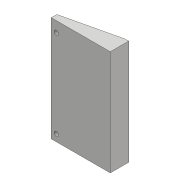
# Autodesk Inventor part: Buck_Bracket
Saved by Autodesk Inventor 2018 (Build 220112000, 112)
## iProperties
Created: 2019-11-08
Part Number: Buck_Bracket
Material: Generic
Document SubType Name: Modeling
Designer: Clevo
Density: 1 g/cm^3
Appearance: Default
Author: Clevo
Autodesk Inventor part; units mm, degrees
ref_plane "YZ Plane" through (0, 0, 0) normal (1, 0, 0) x (0, 1, 0)
ref_plane "XZ Plane" through (0, 0, 0) normal (0, 1, 0) x (-1, 0, 0)
ref_plane "XY Plane" through (0, 0, 0) normal (0, 0, 1) x (1, 0, 0)
sketch "Sketch1" plane through (0, 0, 0) normal (0, 1, 0) x (-1, 0, 0)
  line L0 (-15, -27.5) -> (15, -27.5)
  line L1 (15, -27.5) -> (15, 27.5)
  line L2 (15, 27.5) -> (-15, 27.5)
  line L3 (-15, 27.5) -> (-15, -27.5)
  line L4 (-15, -27.5) -> (15, 27.5) construction
  line L5 (15, -27.5) -> (-15, 27.5) construction
  point P0 (0, 0)
  dimension "d0" = 55
  dimension "d1" = 30
  constraints: 12 end point, 2 midpoint, 2 parallel, 1 horizontal, 1 perpendicular
  measures "d0" distance of L0.end L1.end
  measures "d1" distance of L0.start L0.end
extrude "Extrusion1" add sketch "Sketch1" along normal blind 3
sketch "Sketch2" plane through (0, 3, 0) normal (0, 1, 0) x (1, 0, 0)
  line L0 (10.75, 21.75) -> (-10.75, 21.75)
  line L1 (-10.75, 21.75) -> (-10.75, -21.75)
  line L2 (-10.75, -21.75) -> (10.75, -21.75)
  line L3 (10.75, -21.75) -> (10.75, 21.75)
  line L4 (10.75, 21.75) -> (-10.75, -21.75) construction
  line L5 (-10.75, 21.75) -> (10.75, -21.75) construction
  point P0 (0, 0)
  dimension "d4" = 43.5
  dimension "d5" = 21.5
  constraints: 12 end point, 2 midpoint, 2 parallel, 1 horizontal, 1 perpendicular
  measures "d4" distance of L0.end L1.end
  measures "d5" distance of L1.end L2.end
extrude "Extrusion2" cut sketch "Sketch2" against normal blind 1.6
sketch "Sketch3" plane through (15, 0, 27.5) normal (1, 0, 0) x (0, 0, -1)
  line L0 (55, 0) -> (0, 0) projected
  line L1 (0, 0) -> (55, 0)
  line L2 (55, 0) -> (55, 10)
  line L3 (55, 10) -> (0, 10)
  line L4 (0, 10) -> (0, 0)
  line L5 (55, 0) -> (55, 3) projected
  point P0 (27.5, 0)
  dimension "d8" = 10
  constraints: 8 end point, 2 parallel, 1 collinear, 1 horizontal, 1 perpendicular
  measures "d8" distance of L3.end L0.end
extrude "Extrusion3" add sketch "Sketch3" along normal blind 2
sketch "Sketch4" plane through (-15, 0, 27.5) normal (0, 0, 1) x (1, 0, 0)
  line L0 (0, 0) -> (32, 0) projected
  line L1 (32, 10) -> (32, 0) projected
  line L2 (30, 10) -> (32, 10) projected
  line L3 (30, 10) -> (30, 3) projected
  line L4 (0, 3) -> (30, 3) projected
  line L5 (0, 0) -> (0, 3) projected
  line L6 (0, 3) -> (30, 3) projected
  line L7 (30, 10) -> (32, 10) projected
  line L8 (0, 3) -> (30, 10)
  point P0 (15, 0)
  constraints: 2 end point
extrude "Extrusion4" add sketch "Sketch4" along normal blind 2
sketch "Sketch5" plane through (0, 3, 0) normal (0, 1, 0) x (1, 0, 0)
  line L0 (12.25, 23.75) -> (-12.25, 23.75)
  line L1 (-12.25, 23.75) -> (-12.25, -23.75)
  line L2 (-12.25, -23.75) -> (12.25, -23.75)
  line L3 (12.25, -23.75) -> (12.25, 23.75)
  line L4 (12.25, 23.75) -> (-12.25, -23.75) construction
  line L5 (-12.25, 23.75) -> (12.25, -23.75) construction
  line L6 (-10.75, -21.75) -> (-10.75, 21.75) projected
  line L7 (10.75, -21.75) -> (-10.75, -21.75) projected
  point P0 (0, 0)
  dimension "d13" = 1.5
  dimension "d14" = 2
  constraints: 12 end point, 2 midpoint, 2 parallel, 1 horizontal, 1 perpendicular
  measures "d13" distance between parallel lines of L6 L1
  measures "d14" distance between parallel lines of L2 L7
hole "Hole1" at (-12.25, 3, 23.75) at (-12.25, 3, -23.75) direction (0, -1, 0) diameter 2.459 end through all thread size "M3x0.5" class "6H" standard "ANSI Metric M Profile"
body "Solid1"
